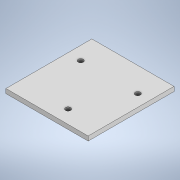
# Autodesk Inventor part: Sensor_Schutzplatte
Saved by Autodesk Inventor 2022.2 (Build 262287010, 287A)
## iProperties
Created: 2024-02-16
Part Number: Sensor_Schutzplatte
Material: Generic
Document SubType Name: Modeling
Designer: ppovolni
Density: 1 g/cm^3
Appearance: Default
Author: ppovolni
Autodesk Inventor part; units mm, degrees
ref_plane "YZ Plane" through (0, 0, 0) normal (1, 0, 0) x (0, 1, 0)
ref_plane "XZ Plane" through (0, 0, 0) normal (0, 1, 0) x (-1, 0, 0)
ref_plane "XY Plane" through (0, 0, 0) normal (0, 0, 1) x (1, 0, 0)
sketch "Skizze1" plane through (0, 0, 0) normal (0, 1, 0) x (-1, 0, 0)
  line L0 (0, 0) -> (-45.5, 0) construction
  line L1 (-45.5, 0) -> (-45.5, -48) construction
  line L2 (-45.5, -48) -> (0, -48) construction
  line L3 (0, -48) -> (0, 0) construction
  circle A0 centre (-4, -36.5) radius 1.75
  circle A1 centre (-42.5, -36.5) radius 1.75
  circle A2 centre (-27.95, -4) radius 1.75
  line L4 (5, -53) -> (-50.5, -53)
  line L5 (-50.5, -53) -> (-50.5, 5)
  line L6 (-50.5, 5) -> (5, 5)
  line L7 (5, 5) -> (5, -53)
  dimension "d0" = 45.5
  dimension "d1" = 48
  dimension "d2" = 11.5
  dimension "d3" = 11.5
  dimension "d4" = 3
  dimension "d5" = 4
  dimension "d6" = 17.55
  dimension "d7" = 4
  dimension "d8" = 3.5
  dimension "d9" = 5
  dimension "d10" = 5
  dimension "d11" = 5
  dimension "d12" = 5
  constraints: 16 end point, 4 parallel, 3 centre point, 2 equal radius, 2 horizontal, 2 perpendicular
  measures "d0" distance of L1.end L2.end
  measures "d1" distance of L2.end L0.start
  measures "d2" distance from line of A0.centre L2
  measures "d3" distance from line of A1.centre L2
  measures "d4" distance from line of L1 A1.centre
  measures "d5" distance from line of L3 A0.centre
  measures "d6" distance from line of L1 A2.centre
  measures "d7" distance from line of L0 A2.centre
  measures "d8" diameter of A0
  measures "d9" distance between parallel lines of L2 L4
  measures "d10" distance between parallel lines of L1 L5
  measures "d11" distance between parallel lines of L6 L0
  measures "d12" distance between parallel lines of L7 L3
extrude "Extrusion1" add sketch "Skizze1" along normal blind 3
